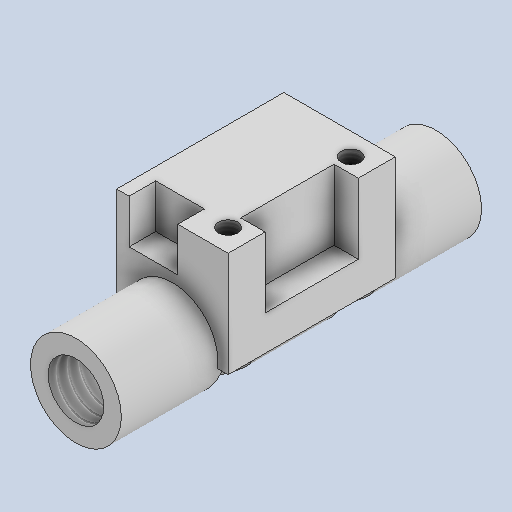
# Autodesk Inventor part: Line Sensor 6 Bracket
Saved by Autodesk Inventor 2024 (Build 280153000, 153)
## iProperties
Created: 2023-10-20
Part Number: Line Sensor 6 Bracket
Material: Generic
Document SubType Name: Modeling
Designer: olson
Density: 1 g/cm^3
Appearance: Default
Author: olson
Autodesk Inventor part; units mm, degrees
ref_plane "YZ Plane" through (0, 0, 0) normal (1, 0, 0) x (0, 1, 0)
ref_plane "XZ Plane" through (0, 0, 0) normal (0, 1, 0) x (-1, 0, 0)
ref_plane "XY Plane" through (0, 0, 0) normal (0, 0, 1) x (1, 0, 0)
sketch "Sketch1" plane through (0, 0, 0) normal (0, 1, 0) x (-1, 0, 0)
  line L0 (0, -55.88) -> (-12.7, -55.88)
  line L1 (-12.7, -36.83) -> (0, -36.83)
  line L2 (0, -36.83) -> (0, -55.88)
  line L3 (-12.7, -55.88) -> (-12.7, -36.83)
  dimension "d1" = 19.05
  dimension "d2" = 12.7
  constraints: 8 end point, 2 perpendicular, 1 horizontal, 1 vertical
  measures "d1" distance of L1.end L0.start
  measures "d2" distance of L0.start L0.end
extrude "Extrusion1" add sketch "Sketch1" along normal blind 1.5
sketch "Sketch2" plane through (0, 1.5, 0) normal (0, 1, 0) x (1, 0, 0)
  line L0 (12.7, 36.83) -> (12.7, 55.88) projected
  line L1 (12.7, 0) -> (10.16, 0)
  circle A0 centre (10.16, 39.37) radius 1.092
  circle A1 centre (10.16, 53.34) radius 1.092
  line L2 (10.16, 53.34) -> (10.16, 39.37)
  point P0 (0, 0)
  dimension "d8" = 2.184
  dimension "d10" = 2.184
  dimension "d71" = 13.97
  constraints: 4 end point, 2 centre point, 1 horizontal, 1 vertical
  measures "d8" diameter of A0
  measures "d10" diameter of A1
  measures "d71" distance of L2.start L2.end
extrude "Extrusion2" cut sketch "Sketch2" against normal blind 1.5
sketch "Sketch5" plane through (0, 0, -36.83) normal (0, 0, 1) x (1, 0, 0)
  line L0 (12.7, 0) -> (0, 0) projected
  line L1 (6.35, 0) -> (6.35, 1.5)
  line L2 (12.7, 1.5) -> (0, 1.5) projected
  line L3 (0, 0) -> (0, 1.5) projected
  line L4 (0, 0.75) -> (12.7, 0.75)
  line L5 (12.7, 0) -> (12.7, 1.5) projected
  circle A0 centre (6.35, 0.75) radius 5.175
  dimension "d30" = 10.35
  constraints: 4 end point, 4 midpoint, 1 centre point
  measures "d30" diameter of A0
extrude "Extrusion5" add sketch "Sketch5" along normal blind 2 contours A0 L0 | L0 L1 L4 A0 | L0 A0 L4 L1 | L4 L1 L2 A0 | L4 A0 L2 L1 | L2 A0
sketch "Sketch6" plane through (6.35, 0.75, -34.83) normal (0, 0, 1) x (1, 0, 0)
  circle A0 centre (0, 0) radius 5.175
  circle A1 centre (0, 0) radius 3.175
  point P0 (-6.35, -0.75)
  dimension "d35" = 6.35
  constraints: 2 centre point, 1 coincident
  measures "d35" diameter of A1
extrude "Extrusion6" add sketch "Sketch6" along normal blind 9
sketch "Sketch7" plane through (12.7, 0, -55.88) normal (0, 0, -1) x (-1, 0, 0)
  line L0 (0, 0) -> (0, 1.5) projected
  line L1 (0, 0.75) -> (12.7, 0.75)
  line L2 (12.7, 0) -> (12.7, 1.5) projected
  line L3 (11.4704, 1.5) -> (1.2296, 1.5) projected
  line L4 (6.35, 1.5) -> (6.35, 0)
  circle A0 centre (6.35, 0.75) radius 5.175
  constraints: 4 end point, 4 midpoint, 1 centre point, 1 perpendicular
extrude "Extrusion7" add sketch "Sketch7" along normal blind 2
sketch "Sketch8" plane through (6.35, 0.75, -57.88) normal (0, 0, -1) x (-1, 0, 0)
  circle A0 centre (0, 0) radius 5.175
  circle A1 centre (0, 0) radius 3.175
  point P0 (6.35, -0.75)
  dimension "d40" = 6.35
  constraints: 2 centre point, 1 coincident
  measures "d40" diameter of A1
extrude "Extrusion8" add sketch "Sketch8" along normal blind 9
thread "Thread1" size "1/4-20 UNC" class "2B" standard "ANSI Unified Screw Threads" full length
thread "Thread2" size "1/4-20 UNC" class "2B" standard "ANSI Unified Screw Threads" full length
sketch "Sketch9" plane through (0, 0, -36.83) normal (0, 0, -1) x (-1, 0, 0)
  arc A0 (-11.4704, 0) -> (-1.2296, 0) centre (-6.35, 0.75) ccw projected
  line L0 (0, 0) -> (-1.2296, 0) projected
  line L1 (-11.4704, 0) -> (-1.2296, 0)
  circle A1 centre (-6.35, 0.75) radius 5.175
  constraints: 2 end point, 1 centre point, 1 coincident, 1 concentric, 1 horizontal
extrude "Extrusion9" add sketch "Sketch9" along normal up to next contours L1 A0
sketch "Sketch10" plane through (10.16, 0, -39.37) normal (0, 1, 0) x (1, 0, 0)
  circle A0 centre (0, 0) radius 1.092
  circle A1 centre (0, 13.97) radius 1.092 projected
  circle A2 centre (0, 13.97) radius 1.092
  point P0 (-10.16, -39.37)
  dimension "d60" = 2.184
  constraints: 2 centre point, 1 coincident
  measures "d60" diameter of A0
extrude "Extrusion10" cut sketch "Sketch10" against normal up to next
sketch "Sketch12" plane through (0, 1.5, 0) normal (0, 1, 0) x (1, 0, 0)
  circle A0 centre (10.16, 39.37) radius 1.092 projected
  circle A1 centre (10.16, 39.37) radius 1.092
  circle A2 centre (10.16, 39.37) radius 2.2225
  circle A3 centre (10.16, 53.34) radius 1.092 projected
  circle A4 centre (10.16, 53.34) radius 1.092
  circle A5 centre (10.16, 53.34) radius 2.2225
  point P0 (0, 0)
  dimension "d54" = 4.445
  dimension "d55" = 4.445
  constraints: 4 centre point, 4 coincident
  measures "d54" diameter of A2
  measures "d55" diameter of A5
extrude "Extrusion11" cut sketch "Sketch12" against normal blind 5.925
sketch "Sketch13" plane through (0, 1.5, 0) normal (0, 1, 0) x (1, 0, 0)
  line L0 (12.7, 36.83) -> (12.7, 55.88) projected
  line L1 (12.7, 55.88) -> (0, 55.88)
  line L2 (0, 55.88) -> (0, 36.83)
  line L3 (12.7, 36.83) -> (12.7, 55.88)
  circle A0 centre (10.16, 53.34) radius 1.092 projected
  circle A1 centre (10.16, 53.34) radius 1.092
  line L4 (10.16, 53.34) -> (10.16, 39.37)
  circle A2 centre (10.16, 39.37) radius 1.092
  line L5 (0, 36.83) -> (12.7, 36.83)
  point P0 (0, 0)
  point P1 (12.7, 0)
  dimension "d72" = 13.97
  dimension "d73" = 2.184
  constraints: 10 end point, 2 centre point, 2 coincident, 2 perpendicular, 1 horizontal, 1 parallel, 1 point on line, 1 vertical
  measures "d72" distance of L4.start L4.end
  measures "d73" diameter of A2
extrude "Extrusion12" add sketch "Sketch13" along normal blind 10.4775 contours L5 L2 L1 L0 | A2
thread "Thread6" size "2-56 UNC" class "2B" standard "ANSI Unified Screw Threads" full length
sketch "Sketch14" plane through (10.16, 1.5, -53.34) normal (0, -1, 0) x (1, 0, 0)
  circle A0 centre (0, 0) radius 1.092 projected
  circle A1 centre (0, 0) radius 2.2225
  circle A2 centre (0, 13.97) radius 2.2225 projected
  circle A3 centre (0, 13.97) radius 2.2225
  circle A4 centre (0, 0) radius 1.092
  circle A5 centre (0, 13.97) radius 1.092
  point P0 (-10.16, 53.34)
  constraints: 4 centre point, 4 coincident, 1 concentric
extrude "Extrusion13" cut sketch "Sketch14" against normal blind 1
sketch "Sketch15" plane through (10.16, 1.5, -39.37) normal (0, -1, 0) x (1, 0, 0)
  circle A0 centre (0, 0) radius 1.092
  point P0 (-10.16, 39.37)
  constraints: 1 centre point
extrude "Extrusion14" cut sketch "Sketch15" against normal through all
thread "Thread7" size "2-56 UNC" class "2B" standard "ANSI Unified Screw Threads" full length
sketch "Sketch16" plane through (0, 11.9775, 0) normal (0, 1, 0) x (1, 0, 0)
  line L0 (11.525, 36.83) -> (1.175, 36.83) projected
  line L1 (3.175, 34.83) -> (9.525, 34.83) projected
  line L2 (1.921, 36.83) -> (6.461, 36.83)
  line L3 (6.461, 36.83) -> (6.961, 36.83)
  line L4 (6.961, 36.83) -> (6.961, 39.854)
  line L5 (6.961, 39.854) -> (1.421, 39.854)
  line L6 (1.421, 39.854) -> (1.421, 36.83)
  line L7 (1.421, 36.83) -> (1.921, 36.83)
  point P0 (0, 0)
  point P1 (0, 36.83)
  point P2 (1.2296, 36.83)
  point P3 (11.4704, 36.83)
  dimension "d114" = 0.5
  dimension "d115" = 3.024
  dimension "d116" = 5.54
  constraints: 12 end point, 4 point on line, 3 perpendicular, 1 collinear
  measures "d114" distance of L2.end L3.end
  measures "d115" distance of L3.end L4.end
  measures "d116" distance of L4.end L5.end
extrude "Extrusion15" cut sketch "Sketch16" against normal blind 5
sketch "Sketch17" plane through (0, 11.9775, 0) normal (0, 1, 0) x (1, 0, 0)
  line L0 (12.7, 36.83) -> (12.7, 55.88) projected
  line L1 (12.7, 55.88) -> (0, 55.88) projected
  line L2 (0, 36.83) -> (12.7, 36.83) projected
  line L3 (0, 36.83) -> (12.7, 36.83)
  line L4 (12.7, 36.83) -> (12.7, 55.88)
  line L5 (12.7, 55.88) -> (0, 55.88)
  line L6 (0, 55.88) -> (0, 36.83)
  line L7 (11.4704, 41.1651) -> (11.4704, 51.5449) projected
  line L8 (11.43, 42.545) -> (12.43, 42.545) construction
  line L9 (11.43, 50.165) -> (12.43, 50.165) construction
  line L10 (12.7, 41.545) -> (12.7, 51.165)
  line L11 (12.7, 41.545) -> (12.7, 41.045)
  line L12 (12.7, 41.045) -> (9.93, 41.045)
  line L13 (9.93, 41.045) -> (9.93, 51.665)
  line L14 (9.93, 51.665) -> (12.7, 51.665)
  line L15 (12.7, 51.165) -> (12.7, 51.665)
  point P0 (0, 0)
  dimension "d110" = 2.77
  dimension "d111" = 10.62
  dimension "d112" = 90
  constraints: 24 end point, 4 perpendicular, 4 point on line, 3 horizontal, 2 parallel
  measures "d110" distance of L11.end L12.end
  measures "d111" distance of L12.end L13.end
  measures "d112" angle of L12 L13
extrude "Extrusion16" cut sketch "Sketch17" against normal blind 8 contours L12 L13 L14 L0
body "Solid1"
